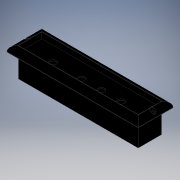
# Autodesk Inventor part: Bessel
Saved by Autodesk Inventor 2017 (Build 210142000, 142)
## iProperties
Created: 2019-01-31
Part Number: Bessel
Material: Generic
Document SubType Name: Modeling
Designer: Mitch
Density: 1 g/cm^3
Appearance: Black
Author: Mitch
Autodesk Inventor part; units mm, degrees
ref_plane "YZ Plane" through (0, 0, 0) normal (1, 0, 0) x (0, 1, 0)
ref_plane "XZ Plane" through (0, 0, 0) normal (0, 1, 0) x (-1, 0, 0)
sketch "Sketch1" plane through (0, 0, 0) normal (0, 1, 0) x (-1, 0, 0)
  line L0 (0, 0) -> (-130.81, 0)
  line L1 (-130.81, 0) -> (-130.81, -25.4)
  line L2 (-130.81, -25.4) -> (0, -25.4)
  line L3 (0, -25.4) -> (0, 0)
  dimension "d0" = 130.81
  dimension "d1" = 25.4
  constraints: 8 end point, 2 parallel, 1 horizontal, 1 perpendicular
  measures "d0" distance of L2.end L1.end
  measures "d1" distance of L1.end L0.end
extrude "Extrusion1" add sketch "Sketch1" along normal blind 25.4
shell "Shell1" thickness 1.27 removed faces 1 at (87.2067, 0, -8.4667)
sketch "Sketch2" plane through (0, 25.4, 0) normal (0, 1, 0) x (1, 0, 0)
  circle A0 centre (28.549, 9.295) radius 3 projected
  circle A1 centre (59.5104, 9.295) radius 3 projected
  circle A2 centre (81.1754, 9.295) radius 3 projected
  circle A3 centre (102.8404, 9.295) radius 3 projected
  circle A4 centre (28.549, 9.295) radius 3.556
  circle A5 centre (59.5104, 9.295) radius 3.556
  circle A6 centre (81.1754, 9.295) radius 3.556
  circle A7 centre (102.8404, 9.295) radius 3.556
  point P0 (0, 0)
  dimension "d5" = 7.112
  dimension "d6" = 7.112
  dimension "d7" = 7.112
  dimension "d8" = 7.112
  constraints: 4 centre point, 4 coincident
  measures "d5" diameter of A4
  measures "d6" diameter of A5
  measures "d7" diameter of A6
  measures "d8" diameter of A7
extrude "Extrusion2" cut sketch "Sketch2" against normal blind 25.4 contours A0 | A1 | A2 | A3 | A4 | A5 | A6 | A7
sketch "Sketch3" plane through (0, 25.4, 0) normal (0, 1, 0) x (1, 0, 0)
  circle A0 centre (81.1754, 9.295) radius 3.556 projected
  circle A1 centre (28.549, 9.295) radius 3.556 projected
  circle A2 centre (59.5104, 9.295) radius 3.556 projected
  circle A3 centre (102.8404, 9.295) radius 3.556 projected
  line L0 (0, 0) -> (130.81, 0) projected
  line L1 (130.81, 0) -> (130.81, 25.4) projected
  line L2 (130.81, 25.4) -> (0, 25.4) projected
  line L3 (0, 25.4) -> (0, 0) projected
  line L4 (-6.35, 31.75) -> (137.16, 31.75)
  line L5 (137.16, 31.75) -> (137.16, -6.35)
  line L6 (137.16, -6.35) -> (-6.35, -6.35)
  line L7 (-6.35, -6.35) -> (-6.35, 31.75)
  dimension "d11" = 6.35
  constraints: 8 end point, 3 other
  measures "d11" distance between parallel lines of L2 L4
extrude "Extrusion3" add sketch "Sketch3" along normal blind 6.35 contours L4 L5 L6 L7
fillet "Fillet1" radius 5.842 4 edges at (-6.35, 31.75, -12.7) (65.405, 31.75, -31.75) (65.405, 31.75, 6.35) (137.16, 31.75, -12.7)
ref_plane "Work Plane1" through (0, 31.75, 0) normal (0, -1, 0) x (1, 0, 0)
sketch "Sketch4" plane through (0, 31.75, 0) normal (0, -1, 0) x (1, 0, 0)
  line L0 (0, -25.4) -> (0, 0) projected
  line L1 (0, 0) -> (130.81, 0) projected
  line L2 (130.81, 0) -> (130.81, -25.4) projected
  line L3 (130.81, -25.4) -> (0, -25.4) projected
  line L4 (-6.35, -31.75) -> (137.16, -31.75) projected
  line L5 (137.16, -31.75) -> (137.16, 6.35) projected
  line L6 (137.16, 6.35) -> (-6.35, 6.35) projected
  line L7 (-6.35, 6.35) -> (-6.35, -31.75) projected
  point P0 (-3.175, -12.7)
  point P1 (133.985, -12.7)
  dimension "d25" = 19.05
  dimension "d26" = 3.175
  dimension "d27" = 19.05
  dimension "d28" = 3.175
  measures "d25" distance from line of L4 point (-3.175, -12.7)
  measures "d26" distance from line of L7 point (-3.175, -12.7)
  measures "d27" distance from line of L4 point (133.985, -12.7)
  measures "d28" distance from line of L5 point (133.985, -12.7)
hole "Hole2" at (-3.175, 31.75, -12.7) at (133.985, 31.75, -12.7) direction (0, -1, 0) diameter 2.794 end through all counterbore diameter 5.1562 counterbore depth 3.175 clearance for "Socket Head Cap Screw" size "#3" standard "Ansi Unified Screw Threads"
body "Solid1"
